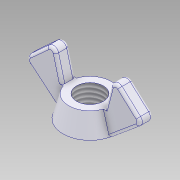
# Autodesk Inventor part: Гайка-барашек М5
Saved by Autodesk Inventor 2018 (Build 220112000, 112)
## iProperties
Created: 2020-03-18
Part Number: Гайка-барашек М5
Material: Типовые
Document SubType Name: Modeling
Designer: Leancher
Density: 1 g/cm^3
Appearance: По умолчанию
Author: Leancher
Autodesk Inventor part; units mm, degrees
ref_plane "YZ Plane" through (0, 0, 0) normal (1, 0, 0) x (0, 1, 0)
ref_plane "XZ Plane" through (0, 0, 0) normal (0, 1, 0) x (-1, 0, 0)
ref_plane "XY Plane" through (0, 0, 0) normal (0, 0, 1) x (1, 0, 0)
sketch "Эскиз1" plane through (0, 0, 0) normal (0, 1, 0) x (-1, 0, 0)
  line L0 (-2.5, 4) -> (-2.5, 0)
  line L1 (-5, 0) -> (-2.5, 0)
  line L2 (-5, 0) -> (-3.9282, 4)
  line L3 (-2.5, 4) -> (-3.9282, 4)
  line L4 (0, 0) -> (0, 7.6417) construction
  constraints: 10 end point
revolve "Вращение1" add sketch "Эскиз1" angle 360 about axis through (0, 0, 0) along (0, 0, 1)
sketch "Эскиз2" plane through (0, 0, 0) normal (0, 1, 0) x (-1, 0, 0)
  line L0 (-6.7216, 8.8894) -> (-10.15, 5.7727)
  line L1 (-5, 0) -> (-10.1175, 4.2646)
  line L2 (-3.9282, 4) -> (-5.0816, 8.4029)
  arc A0 (-5.0816, 8.4029) -> (-6.7216, 8.8894) centre (-6.049, 8.1495) ccw
  arc A1 (-10.15, 5.7727) -> (-10.1175, 4.2646) centre (-9.4773, 5.0328) ccw
  line L3 (0, 0) -> (0, 6.5882) construction
  line L4 (6.7216, 8.8894) -> (10.15, 5.7727)
  line L5 (5, 0) -> (10.1175, 4.2646)
  line L6 (3.9282, 4) -> (5.0816, 8.4029)
  arc A2 (6.7216, 8.8894) -> (5.0816, 8.4029) centre (6.049, 8.1495) ccw
  arc A3 (10.1175, 4.2646) -> (10.15, 5.7727) centre (9.4773, 5.0328) ccw
  line L7 (-3.9282, 4) -> (-3.4282, 4)
  line L8 (-3.4282, 4) -> (-4.5049, 0)
  line L9 (-4.5049, 0) -> (-5, 0)
  line L10 (3.9282, 4) -> (3.4282, 4)
  line L11 (3.4282, 4) -> (4.5049, 0)
  line L12 (4.5049, 0) -> (5, 0)
  constraints: 26 end point, 11 symmetric about line, 8 point on circle, 4 centre point, 4 tangent, 1 equal radius, 2 other
extrude "Выдавливание1" add sketch "Эскиз2" along normal mid plane 2.5
fillet "Сопряжение1" radius 0.5 20 edges at (5.7646, -1.25, 9.1082) (8.4358, -1.25, 7.3311) (10.4771, -1.25, 5.0113) (7.5587, -1.25, 2.1323) (4.5049, -1.25, 6.2014) (10.4771, 1.25, 5.0113) (7.5587, 1.25, 2.1323) (5.7646, 1.25, 9.1082) (4.5049, 1.25, 6.2014) (8.4358, 1.25, 7.3311) (-5.7646, -1.25, 9.1082) (-8.4358, -1.25, 7.3311) (-10.4771, -1.25, 5.0113) (-7.5587, -1.25, 2.1323) (-4.5049, -1.25, 6.2014) (-5.7646, 1.25, 9.1082) (-8.4358, 1.25, 7.3311) (-10.4771, 1.25, 5.0113) (-7.5587, 1.25, 2.1323) (-4.5049, 1.25, 6.2014)
thread "Резьба1" size "M5x0.8" class "6H" standard "ANSI Metric M Profile" full length
